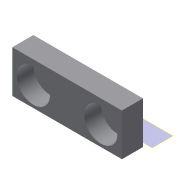
# Autodesk Inventor part: 20_Cube_Insert_Felxuremanipulator_zonly_fiberlid
Saved by Autodesk Inventor 2019.4 (Build 234330000, 330)
## iProperties
Created: 2021-08-17
Part Number: 20_Cube_Insert_Felxuremanipulator_zonly_fiberlid
Material: Generic
Document SubType Name: Modeling
Designer: diederichbenedict
Density: 1 g/cm^3
Appearance: Default
Author: diederichbenedict
Autodesk Inventor part; units mm, degrees
ref_plane "YZ Plane" through (0, 0, 0) normal (1, 0, 0) x (0, 1, 0)
ref_plane "XZ Plane" through (0, 0, 0) normal (0, 1, 0) x (-1, 0, 0)
ref_plane "XY Plane" through (0, 0, 0) normal (0, 0, 1) x (1, 0, 0)
ref_plane "Work Plane1" through (0, -9.3006, 0) normal (0, -1, 0) x (1, 0, 0)
sketch "Sketch1" plane through (0, -9.3006, 0) normal (0, -1, 0) x (1, 0, 0)
  line L0 (8, -4.5373) -> (-18, -4.5373) projected
  line L1 (8, 0) -> (8, -4.5373) projected
  line L2 (8, 0) -> (-18, 0) projected
  line L3 (-18, -4.5373) -> (-18, 0) projected
  line L4 (-18, 6.1006) -> (8, 6.1006)
  line L5 (8, 6.1006) -> (8, 1.1006)
  line L6 (8, 1.1006) -> (-18, 1.1006)
  line L7 (-18, 1.1006) -> (-18, 6.1006)
  line L8 (-8.5, 0.1006) -> (-1.5, 0.1006)
  line L9 (-1.5, 0.1006) -> (-1.5, 1.1006)
  line L10 (-1.5, 1.1006) -> (-8.5, 1.1006)
  line L11 (-8.5, 1.1006) -> (-8.5, 0.1006)
  line L12 (-8.5, 0.1006) -> (-1.5, 1.1006) construction
  line L13 (-1.5, 0.1006) -> (-8.5, 1.1006) construction
  point P0 (0, 0)
  point P1 (-5, 0.6006)
  dimension "d0" = 5
  dimension "d1" = 7
  dimension "d2" = 1
  dimension "d3" = 0
  constraints: 20 end point, 4 parallel, 2 horizontal, 2 midpoint, 2 perpendicular
  measures "d0" distance of L4.end L5.end
  measures "d1" distance of L10.end L9.end
  measures "d2" distance of L9.end L8.end
  measures "d3" distance between parallel lines of L6 L10
extrude "Extrusion1" add sketch "Sketch1" against normal blind 10 contours L4 L5 L6 L7 | L6 L9 L8 L11
sketch "Sketch2" plane through (-18, -9.3006, 6.1006) normal (0, 0, 1) x (1, 0, 0)
  circle A0 centre (5, 4.6503) radius 3.95 projected
  circle A1 centre (21, 4.6503) radius 3.95 projected
  point P0 (18, 9.3006)
extrude "Extrusion2" cut sketch "Sketch2" against normal blind 4
sketch "Sketch3" plane through (8, -9.3006, 6.1006) normal (1, 0, 0) x (0, 0, -1)
  line L0 (6, 0) -> (5, 0) projected
  line L1 (6, 0) -> (6, 10) projected
  line L2 (5, 10) -> (6, 10) projected
  line L3 (5, 0) -> (5, 10) construction
  line L4 (5, 0) -> (6, 5)
  line L5 (6, 0) -> (6, 10) projected
  line L6 (5, 0) -> (5, 10) construction
  line L7 (5, 10) -> (6, 5)
  point P0 (6.1006, 9.3006)
  constraints: 4 end point, 1 midpoint
extrude "Extrusion3" cut sketch "Sketch3" against normal through all
body "Solid1"
